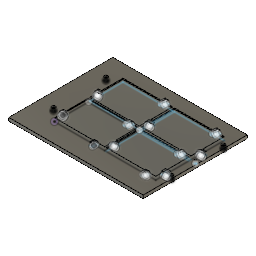
RobotBedAndFrame v49 (Autodesk Fusion 360 design; units mm, degrees)
Autodesk Fusion 360 part; units mm, degrees
sketch "main" plane through (0, 0, 0) normal (0, 0, 1) x (1, 0, 0)
  line L0 (0, 0) -> (128.96, 0)
  line L1 (128.96, 0) -> (128.96, 86.67)
  line L2 (128.96, 86.67) -> (0, 86.67)
  circle A0 centre (-25, 22.7) radius 2.5
  circle A1 centre (277, 22.7) radius 2.5
  circle A2 centre (-25, 157.3) radius 2.5
  circle A3 centre (277, 157.3) radius 2.5
  circle A4 centre (-25, 22.7) radius 4.75
  circle A5 centre (277, 22.7) radius 4.75
  circle A6 centre (-25, 157.3) radius 4.75
  circle A7 centre (277, 157.3) radius 4.75
  line L3 (-0.5342, 30) -> (-0.5342, 20)
  line L4 (-0.5342, 20) -> (-4.0742, 20)
  line L5 (-4.0742, 30) -> (-0.5342, 30)
  line L6 (-4.0742, 20) -> (-4.0742, 30)
  line L7 (132.5, 0) -> (260.26, 0)
  line L8 (132.5, 85.47) -> (132.5, 0)
  line L9 (260.26, 85.47) -> (132.5, 85.47)
  line L10 (260.26, 0) -> (260.26, 85.47)
  line L11 (0, 90.5) -> (127.76, 90.5)
  line L12 (127.76, 175.97) -> (0, 175.97)
  line L13 (127.76, 90.5) -> (127.76, 175.97)
  line L14 (132.5, 90.5) -> (260.26, 90.5)
  line L15 (132.5, 175.97) -> (132.5, 90.5)
  line L16 (260.26, 175.97) -> (132.5, 175.97)
  circle A8 centre (103.96, -2.5174) radius 1.5875
  circle A9 centre (-2.3042, 25) radius 1.5875
  line L17 (98.96, -0.6024) -> (108.96, -0.6024)
  line L18 (108.96, -0.6024) -> (108.96, -4.4324)
  line L19 (108.96, -4.4324) -> (98.96, -4.4324)
  line L20 (98.96, -4.4324) -> (98.96, -0.6024)
  line L21 (98.96, -0.6024) -> (108.96, -4.4324) construction
  line L22 (108.96, -0.6024) -> (98.96, -4.4324) construction
  line L23 (108.96, -8.2624) -> (98.96, -8.2624)
  line L24 (98.96, -4.4324) -> (108.96, -4.4324)
  line L25 (98.96, -8.2624) -> (98.96, -4.4324)
  line L26 (108.96, -4.4324) -> (108.96, -8.2624)
  circle A10 centre (103.96, -6.3474) radius 1.5875
  line L27 (108.96, -0.6024) -> (98.96, -0.6024)
  line L28 (98.96, 3.2276) -> (108.96, 3.2276)
  line L29 (98.96, -0.6024) -> (98.96, 3.2276)
  line L30 (108.96, 3.2276) -> (108.96, -0.6024)
  circle A11 centre (103.96, 1.3126) radius 1.5875
  line L31 (241.46, -8.2624) -> (231.46, -8.2624)
  line L32 (231.46, 3.2276) -> (241.46, 3.2276)
  line L33 (231.46, -0.6024) -> (231.46, 3.2276)
  line L34 (241.46, 3.2276) -> (241.46, -0.6024)
  line L35 (241.46, -0.6024) -> (241.46, -4.4324)
  line L36 (241.46, -4.4324) -> (231.46, -4.4324)
  line L37 (231.46, -4.4324) -> (231.46, -0.6024)
  line L38 (231.46, -8.2624) -> (231.46, -4.4324)
  line L39 (241.46, -4.4324) -> (241.46, -8.2624)
  circle A12 centre (236.46, -2.5174) radius 1.5875
  circle A13 centre (236.46, 1.3126) radius 1.5875
  line L40 (241.46, -0.6024) -> (231.46, -0.6024)
  line L41 (107.76, 80.44) -> (97.76, 80.44)
  line L42 (97.76, 95.53) -> (107.76, 95.53)
  line L43 (97.76, 90.5) -> (97.76, 95.53)
  line L44 (107.76, 95.53) -> (107.76, 90.5)
  line L45 (107.76, 90.5) -> (107.76, 85.47)
  line L46 (107.76, 85.47) -> (97.76, 85.47)
  line L47 (97.76, 85.47) -> (97.76, 90.5)
  line L48 (97.76, 80.44) -> (97.76, 85.47)
  line L49 (107.76, 85.47) -> (107.76, 80.44)
  circle A14 centre (102.76, 87.985) radius 1.5875
  line L50 (107.76, 90.5) -> (97.76, 90.5)
  line L51 (240.26, 80.44) -> (230.26, 80.44)
  line L52 (230.26, 95.53) -> (240.26, 95.53)
  line L53 (230.26, 90.5) -> (230.26, 95.53)
  line L54 (240.26, 95.53) -> (240.26, 90.5)
  line L55 (240.26, 90.5) -> (240.26, 85.47)
  line L56 (240.26, 85.47) -> (230.26, 85.47)
  line L57 (230.26, 85.47) -> (230.26, 90.5)
  line L58 (230.26, 80.44) -> (230.26, 85.47)
  line L59 (240.26, 85.47) -> (240.26, 80.44)
  circle A15 centre (235.26, 87.985) radius 1.5875
  circle A16 centre (235.26, 93.015) radius 1.5875
  line L60 (240.26, 90.5) -> (230.26, 90.5)
  line L61 (107.76, 170.94) -> (97.76, 170.94)
  line L62 (97.76, 186.03) -> (107.76, 186.03)
  line L63 (97.76, 181) -> (97.76, 186.03)
  line L64 (107.76, 186.03) -> (107.76, 181)
  line L65 (107.76, 181) -> (107.76, 175.97)
  line L66 (107.76, 175.97) -> (97.76, 175.97)
  line L67 (97.76, 175.97) -> (97.76, 181)
  line L68 (97.76, 170.94) -> (97.76, 175.97)
  line L69 (107.76, 175.97) -> (107.76, 170.94)
  circle A17 centre (102.76, 178.485) radius 1.5875
  circle A18 centre (102.76, 183.515) radius 1.5875
  line L70 (107.76, 181) -> (97.76, 181)
  line L71 (240.26, 170.94) -> (230.26, 170.94)
  line L72 (230.26, 186.03) -> (240.26, 186.03)
  line L73 (230.26, 181) -> (230.26, 186.03)
  line L74 (240.26, 186.03) -> (240.26, 181)
  line L75 (240.26, 181) -> (240.26, 175.97)
  line L76 (240.26, 175.97) -> (230.26, 175.97)
  line L77 (230.26, 175.97) -> (230.26, 181)
  line L78 (230.26, 170.94) -> (230.26, 175.97)
  line L79 (240.26, 175.97) -> (240.26, 170.94)
  circle A19 centre (235.26, 178.485) radius 1.5875
  circle A20 centre (235.26, 183.515) radius 1.5875
  line L80 (240.26, 181) -> (230.26, 181)
  line L81 (3.0058, 20) -> (-0.5342, 20)
  line L82 (-0.5342, 20) -> (-0.5342, 30)
  line L83 (-0.5342, 30) -> (3.0058, 30)
  line L84 (3.0058, 30) -> (3.0058, 20)
  circle A21 centre (1.2358, 25) radius 1.5875
  line L85 (-4.0742, 20) -> (-7.6142, 20)
  line L86 (-7.6142, 20) -> (-7.6142, 30)
  line L87 (-7.6142, 30) -> (-4.0742, 30)
  line L88 (-4.0742, 30) -> (-4.0742, 20)
  circle A22 centre (-5.8442, 25) radius 1.5875
  line L89 (260.26, 175.97) -> (260.26, 90.5)
  line L90 (123.02, 30) -> (127.76, 30)
  line L91 (137.24, 30) -> (137.24, 20)
  line L92 (127.76, 20) -> (123.02, 20)
  line L93 (132.5, 20) -> (132.5, 30)
  line L94 (137.24, 20) -> (132.5, 20)
  line L95 (132.5, 30) -> (137.24, 30)
  line L96 (127.76, 30) -> (127.76, 20)
  line L97 (127.76, 20) -> (127.76, 30)
  line L98 (123.02, 20) -> (123.02, 30)
  line L99 (127.76, 30) -> (132.5, 30)
  line L100 (132.5, 20) -> (127.76, 20)
  line L101 (132.5, 30) -> (132.5, 20)
  circle A23 centre (130.13, 25) radius 1.5875
  line L102 (255.52, 30) -> (260.26, 30)
  line L103 (269.74, 30) -> (269.74, 20)
  line L104 (260.26, 20) -> (255.52, 20)
  line L105 (265, 20) -> (265, 30)
  line L106 (269.74, 20) -> (265, 20)
  line L107 (265, 30) -> (269.74, 30)
  line L108 (255.52, 20) -> (255.52, 30)
  line L109 (260.26, 30) -> (265, 30)
  line L110 (265, 20) -> (260.26, 20)
  line L111 (265, 30) -> (265, 20)
  circle A24 centre (262.63, 25) radius 1.5875
  line L112 (-7.6142, 120.5) -> (-4.0742, 120.5)
  line L113 (3.0058, 120.5) -> (3.0058, 110.5)
  line L114 (-4.0742, 110.5) -> (-7.6142, 110.5)
  line L115 (-0.5342, 110.5) -> (-0.5342, 120.5)
  line L116 (3.0058, 110.5) -> (-0.5342, 110.5)
  line L117 (-0.5342, 120.5) -> (3.0058, 120.5)
  line L118 (-4.0742, 120.5) -> (-4.0742, 110.5)
  line L119 (-4.0742, 110.5) -> (-4.0742, 120.5)
  line L120 (-7.6142, 110.5) -> (-7.6142, 120.5)
  line L121 (-4.0742, 120.5) -> (-0.5342, 120.5)
  line L122 (-0.5342, 110.5) -> (-4.0742, 110.5)
  line L123 (-0.5342, 120.5) -> (-0.5342, 110.5)
  circle A25 centre (-2.3042, 115.5) radius 1.5875
  line L124 (123.02, 120.5) -> (127.76, 120.5)
  line L125 (137.24, 120.5) -> (137.24, 110.5)
  line L126 (127.76, 110.5) -> (123.02, 110.5)
  line L127 (132.5, 110.5) -> (132.5, 120.5)
  line L128 (137.24, 110.5) -> (132.5, 110.5)
  line L129 (132.5, 120.5) -> (137.24, 120.5)
  line L130 (127.76, 120.5) -> (127.76, 110.5)
  line L131 (127.76, 110.5) -> (127.76, 120.5)
  line L132 (123.02, 110.5) -> (123.02, 120.5)
  line L133 (127.76, 120.5) -> (132.5, 120.5)
  line L134 (132.5, 110.5) -> (127.76, 110.5)
  line L135 (132.5, 120.5) -> (132.5, 110.5)
  circle A26 centre (130.13, 115.5) radius 1.5875
  circle A27 centre (257.89, 115.5) radius 1.5875
  line L136 (255.52, 120.5) -> (260.26, 120.5)
  line L137 (269.74, 120.5) -> (269.74, 110.5)
  line L138 (260.26, 110.5) -> (255.52, 110.5)
  line L139 (265, 110.5) -> (265, 120.5)
  line L140 (269.74, 110.5) -> (265, 110.5)
  line L141 (265, 120.5) -> (269.74, 120.5)
  line L142 (260.26, 120.5) -> (260.26, 110.5)
  line L143 (260.26, 110.5) -> (260.26, 120.5)
  line L144 (255.52, 110.5) -> (255.52, 120.5)
  line L145 (260.26, 120.5) -> (265, 120.5)
  line L146 (265, 110.5) -> (260.26, 110.5)
  line L147 (265, 120.5) -> (265, 110.5)
  circle A28 centre (262.63, 115.5) radius 1.5875
  circle A29 centre (274.4136, 87.985) radius 2.5
  line L148 (0, 0) -> (0, 86.67)
  line L149 (0, 90.5) -> (0, 175.97)
  line L150 (260.26, 30) -> (260.26, 20)
  point P0 (-2.3042, 25)
  point P1 (-2.3042, 30)
  point P2 (-4.0742, 25)
  point P3 (103.96, -2.5174)
  point P4 (236.46, -6.3474)
  point P5 (1.2358, 25)
  point P6 (-5.8442, 25)
  point P7 (-4.0742, 115.5)
  point P8 (1.2358, 115.5)
  point P9 (257.89, 115.5)
  point P10 (0, 87.985)
  point P11 (-5.8442, 115.5)
  dimension "d12" = 128.96
  dimension "d13" = 86.67
  dimension "d61" = 5
  dimension "d69" = 302
  dimension "d70" = 134.6
  dimension "d79" = 22.7
  dimension "d107" = 9.5
  dimension "d145" = 10
  dimension "d151" = 3.54
  dimension "d167" = 90.5
  dimension "d194" = 3.175
  dimension "d205" = 3.175
  dimension "d206" = 20
  dimension "d218" = 10
  dimension "d219" = 3.83
  dimension "d220" = 20
  dimension "d223" = 0
  dimension "d224" = 3.83
  dimension "d227" = 132.5
  dimension "d228" = 90.5
  dimension "d231" = 132.5
  dimension "d232" = 90.5
  dimension "d234" = 5
  dimension "d242" = 260.26
  dimension "d243" = 25
  dimension "d244" = 87.985
  constraint coincident L0.start L148.start
  constraint horizontal L0
  constraint vertical L1
  constraint horizontal L2
  constraint concentric A0 A4
  constraint horizontal L5
  constraint vertical L6
  constraint vertical L3
  constraint coincident L3.end L4.start
  constraint coincident P0 A9.centre
  constraint horizontal L4
  constraint midpoint L5 P1
  constraint vertical P0 P1
  constraint midpoint L6 P2
  constraint horizontal P0 P2
  constraint horizontal L17
  constraint perpendicular L17 L18
  constraint parallel L17 L19
  constraint parallel L18 L20
  constraint coincident L21 P3
  constraint coincident L22 P3
  constraint coincident P3 A8.centre
  constraint perpendicular L16 L89
  constraint horizontal A29.centre P10
  constraint horizontal L12
  constraint perpendicular L2 L148
  constraint perpendicular L12 L149
  constraint vertical L13
  constraint vertical L15
  constraint horizontal L16
  constraint horizontal L7
  constraint vertical L10
  constraint coincident L1 L0.end
  constraint coincident L0.end L1.start
  constraint coincident L7.end L10.start
  constraint coincident L9.start L89
  constraint coincident L0 L7.start
  constraint perpendicular L110 L150
  measures "d12" distance of L0.start L0.end
  measures "d13" distance of L0.start L2.end
  measures "d61" diameter of A0
  measures "d79" vertical distance of L0.start A0.centre
  measures "d107" diameter of A4
  measures "d145" distance of L3.start L3.end
  measures "d151" distance of L5.start L3.start
  measures "d194" diameter of A8
  measures "d205" diameter of A9
  measures "d206" distance of L0.start L4
  measures "d218" distance of L18.end L19.end
  measures "d219" distance of L17.end L18.end
  measures "d220" distance of L1 L18
  measures "d234" diameter of A29
  measures "d242" distance of L0.start L7.end
  measures "d243" horizontal distance of L0.start A0.centre
  measures "d244" distance of L7 A29.centre
sketch "woodBed" plane through (0, 0, 0) normal (0, 0, 1) x (1, 0, 0)
  line L0 (-60, -58) -> (286, -58)
  line L1 (286, -58) -> (286, 210)
  line L2 (286, 210) -> (-60, 210)
  line L3 (-60, 210) -> (-60, -58)
  line L4 (-60, -58) -> (286, 210) construction
  line L5 (286, -58) -> (-60, 210) construction
  point P0 (113, 76)
  point P1 (260.26, 0)
  dimension "d128" = 346
  dimension "d129" = 268
  dimension "d136" = 58
  dimension "d240" = 60
  constraint horizontal L0
  constraint perpendicular L0 L1
  constraint parallel L0 L2
  constraint parallel L1 L3
  constraint coincident L4 P0
  constraint coincident L5 P0
  measures "d128" distance of L1.end L2.end
  measures "d129" distance of L0.end L1.end
  measures "d136" vertical distance of L0.start origin
  measures "d240" distance of L3 origin
extrude "Extrude16" add sketch "woodBed" along normal blind 8.5
extrude "bed FASTENING HOLES" cut sketch "main" along normal blind 9.5 contours A0 | A1 | A2 | A3 | A29
extrude "Extrude24" cut sketch "main" along normal blind 5 from surface at 3.5 contours A4 | A5 | A6 | A7
extrude "slots" cut sketch "main" along normal blind 8.5 from surface at 6 contours L0 L1 L2 L28 L29 L30 L41 L45 L47 L48 L49 L81 L83 L84 L90 L92 L98 L99 L100 L148 | L0 L17 L27 L29 L30 A11 | L81 L83 L84 A21 L148 | L3 L81 L82 L83 A21 L148 | L0 A11 | L0 A11 | A21 L148 | A21 L148 | L1 L96 L97 L99 L100 A23 | L2 L45 L46 L47 A14 | L1 A23 | L7 L8 L9 L10 L32 L33 L34 L51 L58 L59 L91 L94 L95 L102 L104 L108 | L8 L91 L93 L94 L95 L101 | L90 L92 L96 L97 L98 | L2 A14 | L41 L46 L48 L49 | L11 L42 L43 L44 L50 | L11 L12 L13 L42 L43 L44 L61 L68 L69 L113 L116 L117 L124 L126 L132 L149 | L7 L33 L34 A13 L40 | L113 L116 L117 L149 | L115 L116 L117 L123 L149 | L9 L51 L56 L58 L59 | L7 A13 | L7 A13 | L13 L124 L126 L130 L131 L132 | L14 L52 L53 L54 L60 | L14 L15 L16 L52 L53 L54 L71 L78 L79 L89 L125 L128 L129 L136 L138 L144 | L15 L125 L127 L128 L129 L135 | L12 L61 L66 L68 L69 | L89 L136 L138 L142 L143 L144 | L16 L71 L76 L78 L79 | A16 | A27 picked at (128.7391, 25.208) picked at (102.9883, 86.6309)
extrude "Extrude20" cut sketch "main" along normal blind 8.5 contours L19 L23 L24 L25 L26 | L6 L85 L86 L87 L88 | L31 L36 L38 L39 | L112 L114 L118 L119 L120 | L62 L63 L64 L70 | L103 L105 L106 L107 L111 | L137 L139 L140 L141 L147 | L72 L73 L74 L80 | A10 | A18 | A20 | A22
extrude "SHOULDERS" cut sketch "main" along normal blind 5 from surface at 5.61 contours L17 L18 L19 L20 L24 L27 | L3 L4 L5 L6 L82 L88 | L1 L8 L93 L99 L100 L101 A23 | L2 L11 L45 L47 A14 L50 | L1 A23 | L7 L8 L9 L10 L32 L33 L34 L51 L58 L59 L91 L94 L95 L102 L104 L108 | L2 A14 | L11 L12 L13 L42 L43 L44 L61 L68 L69 L113 L116 L117 L124 L126 L132 L149 | L9 L14 L55 L56 L57 L60 | L35 L36 L37 L40 | L115 L118 L119 L121 L122 L123 | L13 L15 L127 L130 L131 L133 L134 L135 | L14 L15 L16 L52 L53 L54 L71 L78 L79 L89 L125 L128 L129 L136 L138 L144 | L12 L65 L66 L67 L70 | L10 L105 L109 L110 L111 L150 | L89 L139 L142 L143 L145 L146 L147 | L16 L75 L76 L77 L80 | A8 | A9 | A12 | A15 | A17 | A19 | A24 | A25 | A26 | A28 picked at (131.3518, 24.7898) picked at (103.042, 87.7796)
extrude "Extrude23" cut sketch "main" along normal blind 8.5 contours L1 A23 | L1 A23 | L2 A14 | L2 A14 | A8 | A9 | A12 | A15 | A17 | A19 | A24 | A25 | A26 | A28
sketch "text" plane through (0, 0, 0) normal (0, 0, 1) x (1, 0, 0)
  line L0 (28.6863, 17.7275) -> (94.7616, 17.7275) construction
  line L1 (94.7616, 17.7275) -> (94.7616, 65.4306) construction
  line L2 (94.7616, 65.4306) -> (28.6863, 65.4306) construction
  line L3 (28.6863, 65.4306) -> (28.6863, 17.7275) construction
  dimension "d134" = 10
equation "opentronsDeckLength = 624.3 mm"
equation "opentronsDeckWidth = 565.2 mm"
equation "slotLength = 132.5 mm"
equation "moduleLength = 127.76 mm + 1.2 mm"
equation "slotWidth = 90.5 mm"
equation "moduleWidth = 85.47 mm + 1.2 mm"
equation "clearance = 10 mm"
equation "d12 = moduleLength"
equation "d13 = moduleWidth"
equation "tubeInternalDiam = 6.86 mm" comment "this is smaller than 4.xx read from code"
equation "xOffset = 14.38 mm"
equation "yOffset = 11.23 mm"
equation "xSpacing = 9 mm"
equation "ySpacing = 9 mm"
equation "labwareHeight = 14.22 mm"
equation "tubeDepth = 10.67 mm"
equation "moduleFasteningScrewHolesDiam = 3.2 mm"
equation "moduleFastenHolesXDistance = 82 mm"
equation "moduleFastenHolesYDistance = 62.3 mm"
equation "d61 = metalFasteningScrewDiamAndPlay"
equation "metalFasteningXGap = 302 mm"
equation "metalFasteningYGap = 134.6 mm"
equation "d69 = metalFasteningXGap"
equation "d70 = metalFasteningYGap"
equation "smallCncMetalBedLenght = 300 mm"
equation "smallCncMetalBedWidth = 180 mm"
equation "d79 = ( smallCncMetalBedWidth - metalFasteningYGap ) / 2"
equation "smallCncBedHeight = 8.5 mm"
equation "moduleFasteningBrassNutHolesDiam = 3.85 mm"
equation "metalFasteningScrewDiamAndPlay = 5 mm"
equation "d107 = metalFastenScrewHeadPocketDiam"
equation "d109 = smallCncBedHeight"
equation "metalFastenScrewHeadPocketDiam = 9.5 mm"
equation "metalFastenScrewHeadPocketHeight = 2.5 mm"
equation "moduleBrassMountHeight = 4.2 mm"
equation "d132 = smallCncBedHeight"
equation "depthOfText = 1.5 mm"
equation "d145 = clipLen"
equation "clipToCorner = 20 mm"
equation "clipLen = 10 mm"
equation "d151 = slotLength - moduleLength"
equation "d166 = -slotLength + moduleLength"
equation "d167 = slotWidth"
equation "d172 = smallCncBedHeight + 1 mm"
equation "d175 = smallCncBedHeight"
equation "d177 = smallCncBedHeight * 0.66"
equation "d194 = clipScrewDiam"
equation "clipScrewDiam = 3.175 mm"
equation "d205 = clipScrewDiam"
equation "d206 = clipToCorner"
equation "d218 = clipLen"
equation "d219 = slotWidth - moduleWidth"
equation "d220 = clipToCorner"
equation "d224 = slotWidth - moduleWidth"
equation "d227 = slotLength"
equation "d228 = slotWidth"
equation "d231 = slotLength"
equation "d232 = slotWidth"
equation "d234 = metalFasteningScrewDiamAndPlay"
equation "d235 = smallCncBedHeight"
equation "d244 = ( 175.97 / 2 ) * 1 mm"
equation "d245 = smallCncBedHeight - metalFastenScrewHeadPocketHeight"
equation "d246 = smallCncBedHeight - 5 mm"
